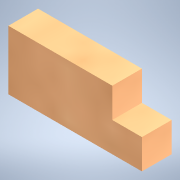
# Autodesk Inventor part: beam2
Saved by Autodesk Inventor 2022 (Build 260153000, 153)
## iProperties
Created: 2021-12-11
Part Number: beam2
Material: Wood (Cherry)
Document SubType Name: Modeling
Designer: dangl
Density: 0.63 g/cm^3
Appearance: Cherry - Natural Low Gloss
Author: dangl
Autodesk Inventor part; units mm, degrees
ref_plane "YZ Plane" through (0, 0, 0) normal (1, 0, 0) x (0, 1, 0)
ref_plane "XZ Plane" through (0, 0, 0) normal (0, 1, 0) x (-1, 0, 0)
ref_plane "XY Plane" through (0, 0, 0) normal (0, 0, 1) x (1, 0, 0)
sketch "Sketch1" plane through (0, 0, 0) normal (0, 0, 1) x (1, 0, 0)
  line L0 (0, -4) -> (0, -2)
  line L1 (-2, 0) -> (-2, -2)
  line L2 (-2, -2) -> (0, -2)
  line L3 (-2, 0) -> (-9, 0)
  line L4 (-9, -2) -> (-9, 0)
  line L5 (-9, -2) -> (-9, -4)
  line L6 (-9, -4) -> (0, -4)
  point P0 (0, 0)
  dimension "d0" = 4
  dimension "d3" = 2
  constraints: 14 end point, 1 horizontal, 1 parallel, 1 perpendicular
  measures "d0" distance of L0.start point (0, 0)
  measures "d3" distance of L0.end L1.end
extrude "Extrusion1" add sketch "Sketch1" along normal blind 2
body "Solid1"
